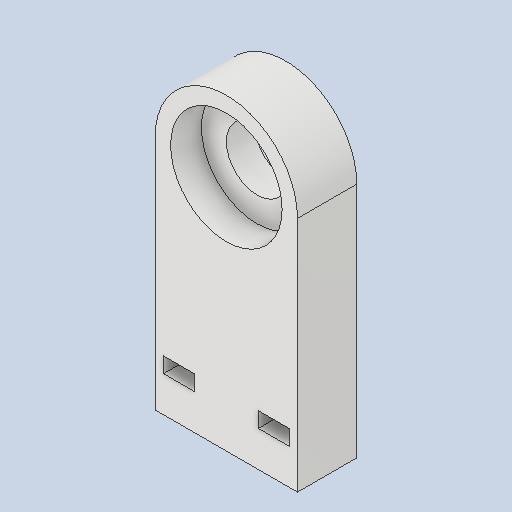
# Autodesk Inventor part: soporte_riel
Saved by Autodesk Inventor 2022 (Build 260153000, 153)
## iProperties
Created: 2019-06-12
Part Number: soporte_riel
Material: Nilón 6/6
Document SubType Name: Modeling
Designer: Usuario
Density: 1.13 g/cm^3
Appearance: Blanco
Author: Usuario
Autodesk Inventor part; units mm, degrees
ref_plane "YZ Plane" through (0, 0, 0) normal (1, 0, 0) x (0, 1, 0)
ref_plane "XZ Plane" through (0, 0, 0) normal (0, 1, 0) x (-1, 0, 0)
ref_plane "XY Plane" through (0, 0, 0) normal (0, 0, 1) x (1, 0, 0)
sketch "Boceto1" plane through (0, 0, 0) normal (0, 0, 1) x (1, 0, 0)
  point P0 (0, 0)
sketch "Boceto2" plane through (0, 0, 0) normal (0, 0, 1) x (1, 0, 0)
  line L0 (0, 0) -> (0, 100)
  line L1 (30, 130) -> (30, 130)
  line L2 (60, 100) -> (60, 0)
  line L3 (60, 0) -> (0, 0)
  arc A0 (30, 130) -> (0, 100) centre (30, 100) ccw
  arc A1 (60, 100) -> (30, 130) centre (30, 100) ccw
  point P0 (0, 130)
  point P1 (60, 130)
  dimension "d1" = 30
  dimension "d2" = 100
  dimension "d3" = 60
  constraints: 8 end point, 4 point on circle, 4 point on line, 4 tangent, 3 perpendicular, 2 centre point, 1 coincident, 1 concentric, 1 vertical
  measures "d1" radius of A0
  measures "d2" distance of L2.start L2.end
  measures "d3" distance of L2.end L0.start
extrude "Extrusión1" add sketch "Boceto2" along normal mid plane 25
sketch "Boceto9" plane through (0, 0, 12.5) normal (0, -1, 0) x (1, 0, 0)
  circle A0 centre (50, -12.5) radius 4
  line L0 (60, -25) -> (0, -25) projected
  circle A1 centre (10, -12.5) radius 4
  line L1 (0, -12.5) -> (60, -12.5) construction
  line L2 (60, 0) -> (60, -25) construction
  line L3 (0, -25) -> (0, 0) construction
  dimension "d52" = 8
  dimension "d88" = 10
  dimension "d89" = 10
  dimension "d90" = 8
  constraints: 2 centre point, 2 end point, 2 point on line, 1 midpoint
  measures "d52" diameter of A0
  measures "d88" distance from line of L3 A1.centre
  measures "d89" distance from line of L2 A0.centre
  measures "d90" diameter of A1
hole "Agujero4" at (10, 0, 0) at (50, 0, 0) direction (0, 1, 0) diameter 8 depth 40
thread "Rosca3" size "M8x1.25" class "6H" standard "ANSI Metric M Profile" full length
thread "Rosca4" size "M8x1.25" class "6H" standard "ANSI Metric M Profile" full length
sketch "Boceto10" plane through (0, 0, 12.5) normal (0, 0, 1) x (1, 0, 0)
  circle A0 centre (30, 100) radius 13
  circle A1 centre (30, 100) radius 23.5125
  line L0 (60, 0) -> (60, 100) projected
  line L1 (0, 100) -> (0, 0) projected
  line L2 (40, 144.843) -> (20, 144.843) projected
  dimension "d64" = 26
  dimension "d65" = 30
  dimension "d68" = 47.025
  dimension "d91" = 100
  constraints: 2 centre point, 1 coincident
  measures "d64" diameter of A0
  measures "d65" distance from line of L0 A1.centre
  measures "d68" diameter of A1
  measures "d91" vertical distance of L0.start A0.centre
extrude "Extrusión5" cut sketch "Boceto10" against normal through all contours A0
extrude "Extrusión6" cut sketch "Boceto10" against normal blind 13
sketch "Boceto12" plane through (0, 0, 12.5) normal (0, 0, 1) x (1, 0, 0)
  line L0 (6, 40) -> (14, 40) construction
  line L1 (10, 40) -> (10, 0) construction
  line L2 (46, 40) -> (54, 40) construction
  line L3 (50, 40) -> (50, 0) construction
  line L4 (0, 0) -> (60, 0) construction
  line L5 (3.4875, 21.5) -> (16.5125, 21.5)
  line L6 (16.5125, 21.5) -> (16.5125, 15)
  line L7 (16.5125, 15) -> (3.4875, 15)
  line L8 (3.4875, 15) -> (3.4875, 21.5)
  line L9 (43.4875, 21.5) -> (56.5125, 21.5)
  line L10 (43.4875, 15) -> (43.4875, 21.5)
  line L11 (56.5125, 15) -> (43.4875, 15)
  line L12 (56.5125, 21.5) -> (56.5125, 15)
  dimension "d92" = 13.025
  dimension "d93" = 6.5125
  dimension "d94" = 15
  dimension "d95" = 6.5
  dimension "d98" = 40
  constraints: 20 end point, 2 horizontal, 2 midpoint, 2 parallel, 2 vertical, 1 perpendicular, 1 point on line, 8 other
  measures "d92" distance of L6.end L7.end
  measures "d93" distance between parallel lines of L1 L6
  measures "d94" distance between parallel lines of L4 L7
  measures "d95" distance of L5.end L6.end
  measures "d98" distance of L5.start L9.start
extrude "Extrusión7" cut sketch "Boceto12" against normal blind 23.0125
